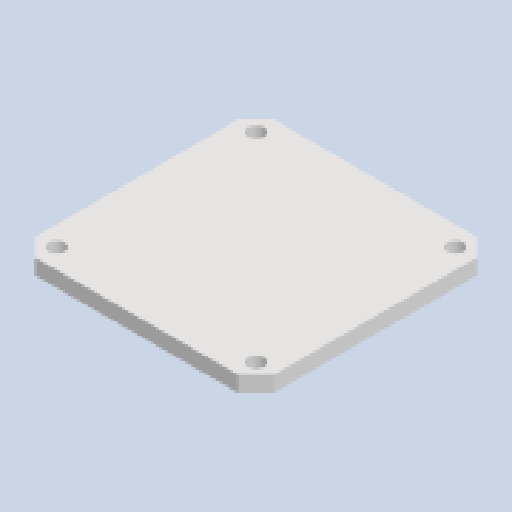
# Autodesk Inventor part: top
Saved by Autodesk Inventor 2025.2 (Build 292293000, 293)
## iProperties
Created: 2025-04-05
Part Number: top
Material: Generic
Document SubType Name: Modeling
Designer: mirewn
Density: 1 g/cm^3
Appearance: Default
Author: mirewn
Autodesk Inventor part; units mm, degrees
ref_plane "YZ Plane" through (0, 0, 0) normal (1, 0, 0) x (0, 1, 0)
ref_plane "XZ Plane" through (0, 0, 0) normal (0, 1, 0) x (-1, 0, 0)
ref_plane "XY Plane" through (0, 0, 0) normal (0, 0, 1) x (1, 0, 0)
sketch "Sketch1" plane through (0, 0, 0) normal (0, 1, 0) x (-1, 0, 0)
  line L0 (25.8285, 25.8285) -> (-25.8285, 25.8285) construction
  line L1 (-25.8285, 25.8285) -> (-25.8285, -25.8285) construction
  line L2 (-25.8285, -25.8285) -> (25.8285, -25.8285) construction
  line L3 (25.8285, -25.8285) -> (25.8285, 25.8285) construction
  line L4 (25.8285, 25.8285) -> (-25.8285, -25.8285) construction
  line L5 (-25.8285, 25.8285) -> (25.8285, -25.8285) construction
  line L6 (31, 26.3139) -> (31, -26.3139)
  line L7 (25.8285, -25.8285) -> (28.6569, -28.6569) construction
  line L8 (28.6569, -28.6569) -> (31, -26.3139)
  line L9 (0, 0) -> (14.4135, 0) construction
  line L10 (25.8285, 25.8285) -> (28.6569, 28.6569) construction
  line L11 (28.6569, 28.6569) -> (31, 26.3139)
  line L12 (-26.3139, 31) -> (26.3139, 31)
  line L13 (28.6569, 28.6569) -> (26.3139, 31)
  line L14 (-28.6569, 28.6569) -> (-26.3139, 31)
  line L15 (-31, -26.3139) -> (-31, 26.3139)
  line L16 (-28.6569, 28.6569) -> (-31, 26.3139)
  line L17 (-28.6569, -28.6569) -> (-31, -26.3139)
  line L18 (26.3139, -31) -> (-26.3139, -31)
  line L19 (-28.6569, -28.6569) -> (-26.3139, -31)
  line L20 (28.6569, -28.6569) -> (26.3139, -31)
  dimension "d0" = 51.657
  dimension "d1" = 51.657
  dimension "d4" = 31
  dimension "d5" = 4
  dimension "d8" = 360
  constraints: 42 end point, 4 coincident, 3 symmetric about line, 2 horizontal, 2 midpoint, 2 parallel, 2 perpendicular, 1 collinear, 1 vertical, 29 other
  measures "d0" distance of L2.end L1.end
  measures "d1" distance of L1.end L0.end
  measures "d4" distance from line of L9.start L6
  measures "d5" distance of L7.start L7.end
extrude "Extrusion1" add sketch "Sketch1" along normal blind 4
hole "Hole1" at (-25.8285, 0, 25.8285) at (-25.8285, 0, -25.8285) at (25.8285, 0, 25.8285) at (25.8285, 0, -25.8285) direction (0, 1, 0) diameter 4.2 end through all
body "Solid1"
